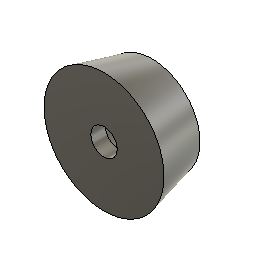
3D Printed Foot 5mm (Autodesk Fusion 360 design; units mm, degrees)
Autodesk Fusion 360 part; units mm, degrees
sketch "Sketch1" plane through (0, 0, 0) normal (0, 1, 0) x (1, 0, 0)
  line L0 (-5, 0) -> (-7.5, -10)
  line L1 (-7.5, -10) -> (5, -10)
  line L2 (5, -10) -> (5, -7)
  line L3 (5, -7) -> (0, -7)
  line L4 (0, -7) -> (0, 0)
  line L5 (-5, 0) -> (0, 0)
  line L6 (5, -10) -> (5, 0.0112) construction
  line L7 (2.25, -7) -> (2.25, -10)
  dimension "d1" = 5
  dimension "d2" = 3
  dimension "d3" = 7
  dimension "d4" = 5
  dimension "d5" = 12.5
  dimension "d8" = 2.75
  measures "d3" distance of L4.end
  measures "d4" distance of L4.end
revolve "Revolve1" add sketch "Sketch1" angle 360 about axis through (5, 0, 10) along (0, 0, -1) contours L0 L1 L3 L4 L5 L7
fillet "Fillet1" [suppressed]
named bodies: "5mm Foot"
